Autodesk Inventor part; units mm, degrees
(part 2 of 2)
sketch "Sketch32" plane through (-14.2515, 5.9336, 0) normal (0, -1, 0) x (1, 0, 0)
  line L0 (0, 0) -> (-3.5381, 0) construction
  line L1 (0, 2.5) -> (0, 0) construction
  line L2 (-10.5381, 2.5) -> (0, 2.5) construction
  line L3 (-10.5381, 2.5) -> (-10.5381, -8) construction
  line L4 (-3.5381, -8) -> (-10.5381, -8) construction
  line L5 (-3.5381, 0) -> (-3.5381, -8) construction
  line L6 (-3.5381, 0) -> (-3.5381, -8) construction
  line L7 (-3.5381, -4) -> (-7.7795, -4) construction
  line L8 (-3.5381, -8) -> (-10.5381, -8) construction
  line L9 (-7.0381, -8) -> (-7.0381, -4) construction
  point P0 (14.2515, 0)
  constraints: 4 end point, 2 midpoint, 1 coincident, 1 horizontal, 1 perpendicular, 1 point on line
hole "Hole3" at (-21.2896, 5.9336, -4) direction (0, 1, 0) diameter 4 end through all countersink diameter 6 countersink angle 90
fillet "Fillet7" radius 2 1 edges at (-17.7896, 7.1836, 0)
fillet "Fillet8" radius 2 4 edges at (-17.7896, 7.1836, -8) (-24.7896, 7.1836, -8) (-24.7896, 7.1836, 2.5) (-14.2515, 5.9336, 1.25)
sketch "Sketch33" plane through (-6.2022, 0, 0) normal (0, 0, -1) x (-1, 0, 0)
  arc A0 (5.3734, 8.4336) -> (9.4475, 3.278) centre (0, 0) ccw projected
  line L0 (0, -10) -> (0, -17)
  line L1 (2.5, -9.6825) -> (2.5, -17)
  line L2 (-2.5, -9.6825) -> (-2.5, -17)
  line L3 (-2.5, -17) -> (2.5, -17)
  point P0 (-6.2022, 0)
  dimension "d140" = 7
  dimension "d141" = 2.5
  dimension "d142" = 2.5
  constraints: 8 end point, 3 point on circle, 2 parallel, 1 horizontal, 1 vertical
  measures "d140" distance of L0.start L0.end
  measures "d141" distance between parallel lines of L0 L1
  measures "d142" distance between parallel lines of L0 L2
extrude "Extrusion23" add sketch "Sketch33" against normal blind 2.5
thicken "Thicken7" operation add thickness 5 both sides no extend neighbours yes toward (0, -1, 0) faces at (-7.0355, -17, 0.8333)
sketch "Sketch36" plane through (-6.2022, 0, 0) normal (0, 0, -1) x (-1, 0, 0)
  line L0 (9.5875, 8.4336) -> (9.5875, 4.9028) construction
  line L1 (9.5875, 8.4336) -> (5.3734, 8.4336) construction
  arc A0 (5.3734, 8.4336) -> (-2.5, -9.6825) centre (0, 0) ccw construction
  line L2 (-2.5, -22) -> (-2.5, -9.6825) construction
  line L3 (2.5, -22) -> (-2.5, -22) construction
  line L4 (2.5, -9.6825) -> (2.5, -22) construction
  arc A1 (2.5, -9.6825) -> (9.4475, 3.278) centre (0, 0) ccw construction
  arc A2 (9.5875, 4.9028) -> (9.4475, 3.278) centre (11.3369, 3.9336) ccw construction
  circle A3 centre (0, 0) radius 3.5 construction
  line L5 (2.5, -22) -> (-2.5, -22) construction
  line L6 (0, -22) -> (0, -13.1272) construction
  line L7 (-1.25, -17) -> (1.25, -17)
  line L8 (1.25, -17) -> (1.25, -22)
  line L9 (1.25, -22) -> (-1.25, -22)
  line L10 (-1.25, -22) -> (-1.25, -17)
  line L11 (-1.25, -17) -> (1.25, -22) construction
  line L12 (1.25, -17) -> (-1.25, -22) construction
  point P0 (-6.2022, 0)
  point P1 (0, -19.5)
  dimension "d160" = 2.5
  dimension "d161" = 5
  constraints: 14 end point, 3 midpoint, 2 parallel, 1 collinear, 1 horizontal, 1 perpendicular, 1 point on line, 1 vertical
  measures "d160" distance of L8.end L9.end
  measures "d161" distance of L7.end L8.end
extrude "Extrusion26" add sketch "Sketch36" along normal blind 3.5
sketch "Sketch37" plane through (-6.2022, 0, -3.5) normal (0, 0, -1) x (-1, 0, 0)
  line L0 (1.25, -17) -> (-1.25, -17) construction
  line L1 (-1.25, -17) -> (-1.25, -22) construction
  line L2 (-1.25, -22) -> (1.25, -22) construction
  line L3 (1.25, -22) -> (1.25, -17) construction
  line L4 (-1.25, -12) -> (1.25, -12)
  line L5 (1.25, -12) -> (1.25, -32.1)
  line L6 (1.25, -32.1) -> (-1.25, -32.1)
  line L7 (-1.25, -32.1) -> (-1.25, -12)
  line L8 (-1.25, -12) -> (1.25, -32.1) construction
  line L9 (1.25, -12) -> (-1.25, -32.1) construction
  point P0 (-6.2022, 0)
  point P1 (0, -22.05)
  dimension "d164" = 2.5
  dimension "d165" = 20.1
  dimension "d166" = 5
  constraints: 12 end point, 2 midpoint, 2 parallel, 1 horizontal, 1 perpendicular
  measures "d164" distance of L5.end L6.end
  measures "d165" distance of L4.end L5.end
  measures "d166" distance between parallel lines of L0 L4
extrude "Extrusion27" add sketch "Sketch37" along normal blind 1.2
sketch "Sketch38" plane through (-6.2022, 0, -4.7) normal (0, 0, -1) x (-1, 0, 0)
  line L0 (1.2416, -12) -> (-1.2584, -12)
  line L1 (-1.2584, -12) -> (-1.2584, -13.2)
  line L2 (-1.2584, -13.2) -> (1.2416, -13.2)
  line L3 (1.2416, -13.2) -> (1.2416, -12)
  line L4 (1.25, -32.1) -> (1.25, -12) projected
  line L5 (1.25, -32.1) -> (-1.25, -32.1)
  line L6 (-1.25, -32.1) -> (-1.25, -30.9)
  line L7 (-1.25, -30.9) -> (1.25, -30.9)
  line L8 (1.25, -30.9) -> (1.25, -32.1)
  line L9 (1.25, -12) -> (-1.25, -12) projected
  point P0 (-6.2022, 0)
  dimension "d169" = 2.5
  dimension "d170" = 1.2
  dimension "d171" = 2.5
  dimension "d172" = 1.2
  constraints: 16 end point, 4 parallel, 2 horizontal, 2 perpendicular, 1 collinear
  measures "d169" distance of L2.end L1.end
  measures "d170" distance of L1.end L0.end
  measures "d171" distance of L6.end L7.end
  measures "d172" distance of L5.end L6.end
extrude "Extrusion28" add sketch "Sketch38" along normal blind 6
thicken "Thicken8" operation add thickness 1.25 both sides no extend neighbours yes toward (1, 0, 0) faces at (-4.9522, -20.3667, -4.3)
thicken "Thicken9" operation add thickness 1.25 both sides no extend neighbours yes toward (1, 0, 0) faces at (-4.9438, -12.4, -6.7)
thicken "Thicken10" operation add thickness 1.25 both sides no extend neighbours yes toward (-1, 0, 0) faces at (-7.4522, -21.6333, -4.3)
thicken "Thicken11" operation add thickness 1.25 both sides no extend neighbours yes toward (-1, 0, 0) faces at (-7.4438, -12.8, -6.7)
fillet "Fillet9" radius 2 5 edges at (-6.2022, -17, -3.5) (-6.2022, -22, 2.5) (-6.2022, -22, -3.5) (-6.2022, -32.1, -3.5) (-6.2022, -12, -3.5)
fillet "Fillet9" radius 1 2 edges at (-6.198, -13.2, -4.7) (-6.2022, -30.9, -4.7)
fillet "Fillet10" radius 2 1 edges at (-6.2022, -17, 0)
sketch "Sketch34" plane through (-6.2022, 0, 0) normal (0, 0, -1) x (-1, 0, 0)
  line L0 (9.5875, 8.4336) -> (9.5875, 4.9028) construction
  line L1 (9.5875, 8.4336) -> (5.3734, 8.4336) construction
  arc A0 (5.3734, 8.4336) -> (-2.5, -9.6825) centre (0, 0) ccw construction
  line L2 (-2.5, -17) -> (-2.5, -9.6825) construction
  line L3 (2.5, -17) -> (-2.5, -17) construction
  line L4 (2.5, -9.6825) -> (2.5, -17) construction
  arc A1 (2.5, -9.6825) -> (9.4475, 3.278) centre (0, 0) ccw construction
  arc A2 (9.5875, 4.9028) -> (9.4475, 3.278) centre (11.3369, 3.9336) ccw construction
  circle A3 centre (0, 0) radius 3.5 construction
  line L5 (-2.5, -17) -> (-2.5, -9.6825) projected
  line L6 (2.5, -9.6825) -> (2.5, -17) projected
  line L7 (-2.5, -17) -> (2.5, -17)
  line L8 (2.5, -17) -> (2.5, -14.5)
  line L9 (2.5, -14.5) -> (-2.5, -14.5)
  line L10 (-2.5, -14.5) -> (-2.5, -17)
  point P0 (-6.2022, 0)
  dimension "d145" = 2.5
  constraints: 8 end point, 2 parallel, 1 horizontal, 1 perpendicular, 1 point on line
  measures "d145" distance of L8.end L7.end
sketch "Sketch35" plane through (-3.7022, -17, -10) normal (0, 0, -1) x (-1, 0, 0)
  line L0 (5, 0) -> (0, 0) projected
  line L1 (5, 0) -> (11.55, 0)
  line L2 (0, 0) -> (-6.55, 0)
  line L3 (-6.55, 0) -> (-7.55, 0)
  line L4 (11.55, 0) -> (12.55, 0)
  line L5 (-7.55, 0) -> (-7.55, 10)
  line L6 (-7.55, 10) -> (-6.55, 10)
  line L7 (-6.55, 10) -> (-6.55, 0)
  line L8 (12.55, 0) -> (12.55, 10)
  line L9 (12.55, 10) -> (11.55, 10)
  line L10 (11.55, 10) -> (11.55, 0)
  line L11 (5, 2.5) -> (0, 2.5) projected
  line L12 (5, 2.5) -> (12.55, 2.5)
  line L13 (0, 2.5) -> (-7.55, 2.5)
  point P0 (-3.7022, 17)
  dimension "d150" = 6.55
  dimension "d151" = 6.55
  dimension "d152" = 18.1
  dimension "d153" = 1
  dimension "d154" = 1
  dimension "d155" = 10
  constraints: 24 end point, 5 perpendicular, 4 horizontal, 3 point on line, 2 vertical
  measures "d150" distance of L0.start L1.end
  measures "d151" distance of L0.end L2.end
  measures "d152" distance of L1.end L2.end
  measures "d153" distance of L2.end L3.end
  measures "d154" distance of L1.end L4.end
  measures "d155" distance of L3.end L5.end
sketch "Sketch26" plane through (-6.2022, 11.2163, 0) normal (-1, 0, 0) x (0, -1, 0)
  line L0 (11.2163, 0) -> (11.2163, 3.9829) construction
  arc A0 (31.3668, -2.1424) -> (21.2163, 2.5) centre (21.2163, -10.918) ccw
  arc A1 (27.7118, -2.1424) -> (21.2163, 0) centre (21.2163, -10.918) ccw
  line L1 (27.7118, -2.1424) -> (31.3668, -2.1424)
  line L2 (21.2163, 0) -> (21.2163, 2.5)
  line L3 (21.2163, 2.5) -> (21.2163, 0)
  dimension "d105" = 2.5
  constraints: 8 end point, 4 point on circle, 2 centre point, 1 vertical
  measures "d105" radial gap between concentric circles of A0 A1
sketch "Sketch27" plane through (-4.7645, 16.4327, -2.1424) normal (0, 0, -1) x (-0.9961947, 0.0871557, 0)
  line L0 (0, 0) -> (0, 3.6549) projected
  arc A0 (2.8644, -0.2506) -> (0, 0) centre (0, -16.4955) ccw projected
  line L1 (3.4991, 3.3488) -> (2.8644, -0.2506) projected
  arc A1 (3.4991, 3.3488) -> (0, 3.6549) centre (0, -16.4955) ccw projected
  line L2 (0, -32.991) -> (0, -36.646) projected
  arc A2 (-2.8644, -32.7404) -> (0, -32.991) centre (0, -16.4955) ccw projected
  line L3 (-3.4991, -36.3398) -> (-2.8644, -32.7404) projected
  arc A3 (-3.4991, -36.3398) -> (0, -36.646) centre (0, -16.4955) ccw projected
  point P0 (-6.1786, -15.955)
sketch "Sketch28" plane through (-17.4522, 11.2163, 0) normal (-1, 0, 0) x (0, -1, 0)
  line L0 (-8.8574, -2.1424) -> (-8.8574, -9.1424) projected
  line L1 (-5.2164, -9.1424) -> (-8.8574, -9.1424) projected
  line L2 (-5.2164, -2.1424) -> (-5.2164, -9.1424) projected
  line L3 (27.6491, -2.1424) -> (27.6491, -9.1424) projected
  line L4 (31.2901, -2.1424) -> (31.2901, -9.1424) projected
  line L5 (31.2901, -9.1424) -> (27.6491, -9.1424) projected
  line L6 (-8.8574, -2.1424) -> (-5.2164, -2.1424)
  line L7 (27.6491, -2.1424) -> (31.2901, -2.1424)
  point P0 (11.2163, 0)
  constraints: 4 end point, 1 collinear, 1 horizontal
sketch "Sketch29" plane through (-17.4522, 11.2163, 0) normal (-1, 0, 0) x (0, 0, 1)
  line L0 (-2.1424, 8.8574) -> (-9.1424, 8.8574) projected
  line L1 (-2.1424, 5.2164) -> (-2.1424, 8.8574) projected
  line L2 (-2.1424, -31.2901) -> (-2.1424, -27.6491) projected
  line L3 (-9.1424, -31.2901) -> (-2.1424, -31.2901) projected
  line L4 (-9.1424, -27.6491) -> (-9.1424, -31.2901) projected
  line L5 (-9.1424, 8.8574) -> (-9.1424, 5.2164) projected
  line L6 (-9.1424, 5.2164) -> (-2.1424, 5.2164) projected
  line L7 (-2.1424, 5.2164) -> (-2.1424, -2.7836)
  line L8 (-2.1424, -2.7836) -> (-9.1424, -2.7836)
  line L9 (-9.1424, -2.7836) -> (-9.1424, 5.2164)
  line L10 (-2.1424, -27.6491) -> (-2.1424, -19.6491)
  line L11 (-2.1424, -19.6491) -> (-9.1424, -19.6491)
  line L12 (-9.1424, -19.6491) -> (-9.1424, -27.6491)
  point P0 (0, -11.2163)
  dimension "d117" = 8
  dimension "d118" = 8
  constraints: 2 end point, 2 point on circle, 1 horizontal
  measures "d117" distance of L1.start L7.end
  measures "d118" distance of L2.end L10.end
sketch "Sketch11" plane through (3.7978, 0, 2.5) normal (0, 1, 0) x (-1, 0, 0)
  line L0 (0, 0) -> (20, 0) construction
  line L1 (10, 0) -> (10, -12) construction
  line L2 (39.9958, -5) -> (39.5, -5) construction
  line L3 (39.9809, -5) -> (39.9958, -5) construction
  line L4 (39.9809, -5) -> (39.9958, -5) construction
  line L5 (35, -3) -> (-15, -3) construction
  line L6 (23.9751, -10.357) -> (23.9751, 0.9681) construction
  arc A0 (23.9751, -3.9751) -> (20, 0) centre (20, -3.9751) ccw
  line L7 (23.9751, -3.9751) -> (23.9751, -12)
  line L8 (0, -2.5) -> (20, -2.5)
  arc A1 (21.4751, -3.9751) -> (20, -2.5) centre (20, -3.9751) ccw
  line L9 (21.4751, -3.9751) -> (21.4751, -12)
  line L10 (0, -2.5) -> (20, -2.5) projected
  line L11 (20, -2.5) -> (20, 0)
  line L12 (20, 0) -> (20, -2.5) projected
  line L13 (21.4751, -12) -> (23.9751, -12)
  point P0 (3.7978, -2.5)
  dimension "d35" = 12
  dimension "d36" = 16.0207
  dimension "d37" = 2.5
  constraints: 14 end point, 4 point on circle, 2 centre point, 2 point on line, 2 vertical, 1 collinear, 1 midpoint, 1 perpendicular, 1 tangent, 2 other
  measures "d35" distance of L1.start L1.end
  measures "d36" distance from line of L6 L2.start
  measures "d37" radial gap between concentric circles of A0 A1
sketch "Sketch18" plane through (-6.2022, 0, -9.5) normal (0, 0, -1) x (-1, 0, 0)
  line L0 (11.4314, -1.0001) -> (13.9219, -1.218) construction
  arc A0 (13.9219, -1.218) -> (13.9219, 1.218) centre (0, 0) ccw construction
  line L1 (11.4314, 1.0001) -> (13.9219, 1.218) construction
  arc A1 (11.4314, -1.0001) -> (11.4314, 1.0001) centre (0, 0) ccw projected
  circle A2 centre (0, 0) radius 3.5 construction
  arc A3 (9.9619, 0.8716) -> (5.7358, 8.1915) centre (0, 0) ccw construction
  arc A4 (5.7358, 8.1915) -> (4.2262, 9.0631) centre (0, 0) ccw construction
  arc A5 (4.2262, 9.0631) -> (-0.8716, -9.9619) centre (0, 0) ccw construction
  arc A6 (-0.8716, -9.9619) -> (0.8716, -9.9619) centre (0, 0) ccw construction
  arc A7 (0.8716, -9.9619) -> (9.9619, -0.8716) centre (0, 0) ccw construction
  arc A8 (9.9619, -0.8716) -> (9.9619, 0.8716) centre (0, 0) ccw construction
  arc A9 (13.9219, -1.218) -> (13.9219, 1.218) centre (0, 0) ccw projected
  line L2 (13.9751, 0) -> (13.9751, 10.6657)
  line L3 (13.9751, 0) -> (13.9751, -11.9219)
  line L4 (11.9751, -13.9219) -> (1.218, -13.9219)
  line L5 (5.9061, 12.6657) -> (11.9751, 12.6657)
  line L6 (4.8496, 10.4) -> (5.9061, 12.6657) projected
  arc A10 (-1.218, -13.9219) -> (1.218, -13.9219) centre (0, 0) ccw projected
  line L7 (-1.0001, -11.4314) -> (-1.218, -13.9219) projected
  arc A11 (6.5818, 9.3998) -> (4.8496, 10.4) centre (0, 0) ccw projected
  arc A12 (-1.0001, -11.4314) -> (1.0001, -11.4314) centre (0, 0) ccw projected
  line L8 (1.0001, -11.4314) -> (10.4314, -11.4314)
  line L9 (9.9619, -0.8716) -> (11.4314, -1.0001) projected
  line L10 (11.4314, -10.4314) -> (11.4314, -1.0001)
  line L11 (11.4314, 1.0001) -> (11.4314, 8.3998)
  line L12 (10.4314, 9.3998) -> (6.5818, 9.3998)
  arc A13 (13.9751, 10.6657) -> (11.9751, 12.6657) centre (11.9751, 10.6657) ccw
  arc A14 (11.9751, -13.9219) -> (13.9751, -11.9219) centre (11.9751, -11.9219) ccw
  arc A15 (10.4314, -11.4314) -> (11.4314, -10.4314) centre (10.4314, -10.4314) ccw
  arc A16 (11.4314, 8.3998) -> (10.4314, 9.3998) centre (10.4314, 8.3998) ccw
  point P0 (-6.2022, 0)
  dimension "d65" = 2
  dimension "d66" = 1
  constraints: 16 end point, 10 point on circle, 8 tangent, 4 centre point, 4 perpendicular, 3 vertical, 2 equal radius, 1 horizontal
  measures "d65" radius of A13
  measures "d66" radius of A15
sketch "Sketch19" plane through (-20.1773, -11.9219, -9.5) normal (-1, 0, 0) x (0, 0, 1)
  line L0 (0, 22.5876) -> (0, 0) projected
  line L1 (0, 0) -> (8, 0) projected
  line L2 (8, 11.9219) -> (8, 0) projected
  line L3 (8, 22.5876) -> (8, 11.9219) projected
  line L4 (0, 22.5876) -> (8, 22.5876) projected
  line L5 (6, 11.9219) -> (6, 2)
  line L6 (6, 2) -> (2, 2)
  line L7 (2, 2) -> (2, 20.5876)
  line L8 (2, 20.5876) -> (6, 20.5876)
  line L9 (6, 20.5876) -> (6, 11.9219)
  point P0 (9.5, 11.9219)
  dimension "d69" = 2
  constraints: 10 end point, 4 other
  measures "d69" distance between parallel lines of L3 L9
sketch "Sketch20" plane through (-18.1773, -13.9219, -9.5) normal (0, -1, 0) x (1, 0, 0)
  line L0 (0, 0) -> (10.7571, 0) projected
  line L1 (10.7571, 0) -> (10.7571, 8) projected
  line L2 (0, 8) -> (10.7571, 8) projected
  line L3 (0, 0) -> (0, 8) projected
  line L4 (8.7571, 2) -> (2, 2)
  line L5 (2, 2) -> (2, 6)
  line L6 (2, 6) -> (8.7571, 6)
  line L7 (8.7571, 6) -> (8.7571, 2)
  point P0 (18.1773, 9.5)
  dimension "d72" = 2
  constraints: 8 end point, 3 other
  measures "d72" distance between parallel lines of L0 L4
sketch "Sketch21" plane through (-20.1773, -11.9219, -9.5) normal (-1, 0, 0) x (0, 0, 1)
  line L0 (2, 20.5876) -> (6, 20.5876) construction
  line L1 (6, 20.5876) -> (6, 2) construction
  line L2 (6, 2) -> (2, 2) construction
  line L3 (2, 2) -> (2, 20.5876) construction
  line L4 (0, 22.5876) -> (0, 0) construction
  line L5 (0, 0) -> (8, 0) construction
  line L6 (8, 11.9219) -> (8, 0) construction
  line L7 (8, 22.5876) -> (8, 11.9219) construction
  line L8 (0, 22.5876) -> (8, 22.5876) construction
  line L9 (0, 22.5876) -> (8, 22.5876)
  line L10 (8, 22.5876) -> (8, 32.5876)
  line L11 (8, 32.5876) -> (0, 32.5876)
  line L12 (0, 32.5876) -> (0, 22.5876)
  line L13 (0, 0) -> (8, 0) projected
  line L14 (0, 0) -> (8, 0)
  line L15 (8, 0) -> (8, -10)
  line L16 (8, -10) -> (0, -10)
  line L17 (0, -10) -> (0, 0)
  point P0 (9.5, 11.9219)
  dimension "d75" = 10
  dimension "d76" = 10
  constraints: 16 end point, 4 parallel, 2 horizontal, 2 perpendicular
  measures "d75" distance of L10.end L9.end
  measures "d76" distance of L14.end L15.end
sketch "Sketch22" plane through (-17.6773, -11.9219, -9.5) normal (1, 0, 0) x (0, 0, -1)
  arc A0 (0, 29.5876) -> (-3, 32.5876) centre (-3, 29.5876) ccw construction
  line L0 (-3, 32.5876) -> (-5, 32.5876) construction
  arc A1 (-5, 32.5876) -> (-8, 29.5876) centre (-5, 29.5876) ccw construction
  line L1 (-8, 29.5876) -> (-8, 24.5876) construction
  line L2 (0, 24.5876) -> (-8, 24.5876) construction
  line L3 (0, 24.5876) -> (0, 29.5876) construction
  arc A2 (-8, -7) -> (-5, -10) centre (-5, -7) ccw construction
  line L4 (-5, -10) -> (-3, -10) construction
  arc A3 (-3, -10) -> (0, -7) centre (-3, -7) ccw construction
  line L5 (0, -7) -> (0, -2) construction
  line L6 (-8, -2) -> (0, -2) construction
  line L7 (-8, -2) -> (-8, -7) construction
  line L8 (-5, -10) -> (-3, -10) construction
  line L9 (-4, -10) -> (-4, -6) construction
  line L10 (-3, 32.5876) -> (-5, 32.5876) construction
  line L11 (-4, 32.5876) -> (-4, 28.5876) construction
  point P0 (-9.5, 11.9219)
  dimension "d80" = 4
  dimension "d81" = 4
  dimension "d90" = 18.1
  dimension "d91" = 1.9051
  dimension "d92" = 2.1009
  constraints: 30 end point, 10 point on line, 5 perpendicular, 4 midpoint, 2 parallel, 1 horizontal
sketch "Sketch24" plane through (-17.6336, -10.4314, -9.5) normal (0, 0, -1) x (-1, 0, 0)
  line L0 (-4.4219, -2) -> (-12.519, -2) projected
  line L1 (-12.519, -2) -> (-12.5589, -2.4558) projected
  arc A0 (-12.5589, -2.4558) -> (-11.5728, -3.543) centre (-11.5627, -2.543) ccw projected
  arc A1 (-11.5728, -3.543) -> (-10.2134, -3.4905) centre (-11.4314, 10.4314) ccw projected
  line L2 (0.0437, -3.4905) -> (-10.2134, -3.4905) projected
  line L3 (0.0437, -8.4905) -> (0.0437, -3.4905) projected
  line L4 (2.5437, -8.4905) -> (0.0437, -8.4905) projected
  line L5 (2.5437, 28.0972) -> (2.5437, -8.4905) projected
  line L6 (0.0437, 28.0972) -> (2.5437, 28.0972) projected
  line L7 (0.0437, 23.0972) -> (0.0437, 28.0972) projected
  line L8 (-4.4219, 23.0972) -> (0.0437, 23.0972) projected
  line L9 (-4.4219, 23.0972) -> (-4.4219, 19.8313) projected
  line L10 (-1, 19.8313) -> (-4.4219, 19.8313) projected
  arc A2 (0, 18.8313) -> (-1, 19.8313) centre (-1, 18.8313) ccw projected
  line L11 (0, 11.4315) -> (0, 18.8313) projected
  arc A3 (0, 9.4313) -> (0, 11.4315) centre (-11.4314, 10.4314) ccw projected
  line L12 (0, 0) -> (0, 9.4313) projected
  arc A4 (-1, -1) -> (0, 0) centre (-1, 0) ccw projected
  line L13 (-4.4219, -1) -> (-1, -1) projected
  line L14 (-4.4219, -1) -> (-4.4219, -2) projected
  line L15 (-4.4219, -1) -> (-4.4219, -3.4905)
  point P0 (-17.6336, 10.4314)
  point P1 (-4.4219, -2)
  constraints: 3 point on line, 2 end point, 1 perpendicular
sketch "Sketch12" plane through (-6.2022, 0, -9.5) normal (0, 0, -1) x (-1, 0, 0)
  circle A0 centre (0, 0) radius 3.5 construction
  line L0 (-1.0001, -11.4314) -> (-1.218, -13.9219) projected
  line L1 (4.8496, 10.4) -> (5.9061, 12.6657) projected
  arc A1 (-1.218, -13.9219) -> (5.9061, 12.6657) centre (0, 0) ccw
  arc A2 (-1.0001, -11.4314) -> (4.8496, 10.4) centre (0, 0) ccw
  point P0 (-6.2022, 0)
  constraints: 4 point on circle, 2 centre point, 2 coincident
sketch "Sketch14" plane through (-11.0518, 10.4, -9.5) normal (0, 0, -1) x (-0.9063078, -0.4226183, 0)
  arc A0 (4.7798, -24.6074) -> (0, 2.5) centre (0, -11.4751) ccw construction
  line L0 (0, 0) -> (0, 2.5) construction
  arc A1 (3.9247, -22.2581) -> (0, 0) centre (0, -11.4751) ccw construction
  line L1 (3.9247, -22.2581) -> (4.7798, -24.6074) construction
  circle A2 centre (0, -11.4751) radius 3.5 construction
  arc A3 (4.7798, -24.6074) -> (0, 2.5) centre (0, -11.4751) ccw projected
  line L2 (12.6708, -5.5798) -> (8.4524, 3.4869)
  line L3 (12.6708, -5.5798) -> (16.8892, -14.6466)
  line L4 (6.1857, 2.4323) -> (10.4041, -6.6344)
  line L5 (10.4041, -6.6344) -> (14.6225, -15.7012)
  line L6 (6.1857, 2.4323) -> (8.4524, 3.4869)
  line L7 (14.6225, -15.7012) -> (16.8892, -14.6466)
  point P0 (-5.6211, -14.0962)
  dimension "d48" = 10
  dimension "d49" = 10
  dimension "d50" = 2.5
  constraints: 12 end point, 1 parallel, 1 point on circle, 1 tangent, 1 other
  measures "d48" distance of L2.start L2.end
  measures "d49" distance of L2.start L3.end
  measures "d50" distance between parallel lines of L2 L4
sketch "Sketch16" plane through (-11.0518, 10.4, -9.5) normal (0, 0, -1) x (-0.9063078, -0.4226183, 0)
  arc A0 (3.9247, -22.2581) -> (0, 0) centre (0, -11.4751) ccw projected
  line L0 (3.9247, -22.2581) -> (4.7798, -24.6074) projected
  arc A1 (4.7798, -24.6074) -> (13.769, -13.8666) centre (0, -11.4751) ccw projected
  line L1 (13.769, -13.8666) -> (14.6225, -15.7012) projected
  line L2 (16.8892, -14.6466) -> (8.4524, 3.4869) projected
  line L3 (6.1857, 2.4323) -> (7.0393, 0.5977) projected
  arc A2 (7.0393, 0.5977) -> (0, 2.5) centre (0, -11.4751) ccw projected
  line L4 (0, 0) -> (0, 2.5) projected
  line L5 (8.4524, 3.4869) -> (6.1857, 2.4323) projected
  line L6 (7.3191, 2.9596) -> (15.7559, -15.1739)
  line L7 (14.6225, -15.7012) -> (16.8892, -14.6466) projected
  line L8 (16.8892, -14.6466) -> (8.4524, 3.4869) projected
  line L9 (7.3191, 2.9596) -> (8.4524, 3.4869)
  line L10 (8.4524, 3.4869) -> (16.8892, -14.6466)
  line L11 (16.8892, -14.6466) -> (15.7559, -15.1739)
  point P0 (-5.6211, -14.0962)
  constraints: 8 end point, 3 centre point, 2 midpoint, 2 perpendicular
sketch "Sketch17" plane through (-20.1687, -10.012, -9.5) normal (-0.9999996, -0.0008594, 0) x (0, 0, 1)
  line L0 (0, 0) -> (0, 20) construction
  line L1 (0, 0) -> (6, 0) construction
  line L2 (6, 10) -> (6, 0) construction
  line L3 (6, 20) -> (6, 10) construction
  line L4 (0, 20) -> (6, 20) construction
  line L5 (0, 20) -> (6, 20) construction
  line L6 (3, 20) -> (3, 0) construction
  line L7 (0, 0) -> (6, 0) construction
  line L8 (3, 20) -> (3, 11.1243) construction
  line L9 (3, 8.8977) -> (3, 0) construction
  point P0 (9.5, 9.9947)
  point P1 (3, 15)
  point P2 (3, 5)
  constraints: 2 end point, 2 midpoint, 2 point on line
body "Solid1"
